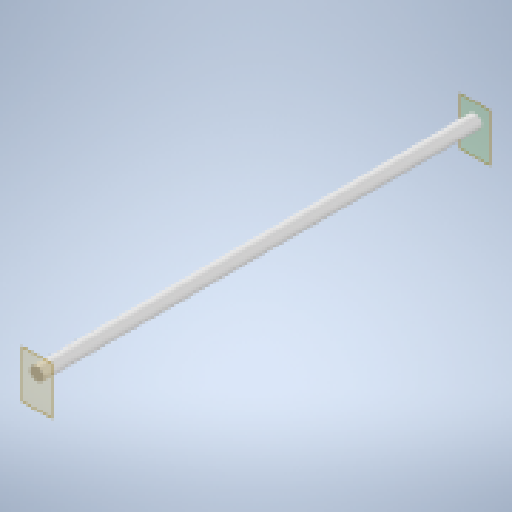
# Autodesk Inventor part: GEAR_SHAFT
Saved by Autodesk Inventor 2024 (Build 280153000, 153)
## iProperties
Created: 2024-04-16
Part Number: GEAR_SHAFT
Material: Generic
Document SubType Name: Modeling
Designer: teeta
Density: 1 g/cm^3
Appearance: Default
Author: teeta
Autodesk Inventor part; units mm, degrees
ref_plane "YZ Plane" through (0, 0, 0) normal (1, 0, 0) x (0, 1, 0)
ref_plane "XZ Plane" through (0, 0, 0) normal (0, 1, 0) x (-1, 0, 0)
ref_plane "XY Plane" through (0, 0, 0) normal (0, 0, 1) x (1, 0, 0)
ref_plane "Work Plane1" through (0, 0, 0) normal (0, 0, 1) x (1, 0, 0)
sketch "Sketch1" plane through (0, 0, 0) normal (0, 0, 1) x (1, 0, 0)
  circle A0 centre (25, 53.553) radius 12.5 projected
  point P0 (0, 0)
ref_plane "Work Plane2" through (50, 0, -809.45) normal (0, 0, -1) x (-1, 0, 0)
extrude "Extrusion1" add sketch "Sketch1" against normal up to surface (809.45 mm away)
body "Solid1"
